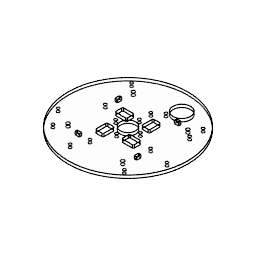
MidPlate_v76 (Autodesk Fusion 360 design; units mm, degrees)
Autodesk Fusion 360 part; units mm, degrees
note: some values were not read from the file. Set by a fixed rule: which face or edge a step refers to.
derive "Sketch1" from "ServoRail v52"
sketch "sketch 220" plane through (0, 0, 0) normal (0, 0, 1) x (1, 0, 0)
  line L0 (-23.75, 13.75) -> (23.75, 13.75) construction
  line L1 (23.75, 13.75) -> (23.75, -13.75) construction
  line L2 (23.75, -13.75) -> (-23.75, -13.75) construction
  line L3 (-23.75, -13.75) -> (-23.75, 13.75) construction
  line L4 (-23.75, 13.75) -> (23.75, -13.75) construction
  line L5 (23.75, 13.75) -> (-23.75, -13.75) construction
  line L6 (-2.75, -24.75) -> (-44.75, -24.75)
  line L7 (-44.75, -24.75) -> (-44.75, -2.75)
  line L8 (-44.75, -2.75) -> (-2.75, -2.75)
  line L9 (-2.75, -2.75) -> (-2.75, -24.75)
  line L10 (-2.75, -24.75) -> (-44.75, -2.75) construction
  line L11 (-44.75, -24.75) -> (-2.75, -2.75) construction
  line L12 (-32.75, -2.75) -> (-32.75, 4.25)
  line L13 (-32.75, 4.25) -> (-29.75, 4.25)
  line L14 (-29.75, 4.25) -> (-29.75, 0.25)
  line L15 (-26.75, 0.25) -> (-26.75, -2.75)
  line L16 (-26.75, 0.25) -> (-29.75, 0.25)
  line L17 (2.75, -44.75) -> (2.75, -2.75)
  line L18 (2.75, -32.75) -> (-4.25, -32.75)
  line L19 (-4.25, -32.75) -> (-4.25, -29.75)
  line L20 (-4.25, -29.75) -> (-0.25, -29.75)
  line L21 (-0.25, -26.75) -> (-0.25, -29.75)
  line L22 (-0.25, -26.75) -> (2.75, -26.75)
  line L23 (24.75, -44.75) -> (2.75, -44.75)
  line L24 (24.75, -2.75) -> (24.75, -44.75)
  line L25 (2.75, -2.75) -> (24.75, -2.75)
  line L26 (44.75, 2.75) -> (2.75, 2.75)
  line L27 (32.75, 2.75) -> (32.75, -4.25)
  line L28 (32.75, -4.25) -> (29.75, -4.25)
  line L29 (29.75, -4.25) -> (29.75, -0.25)
  line L30 (26.75, -0.25) -> (29.75, -0.25)
  line L31 (26.75, -0.25) -> (26.75, 2.75)
  line L32 (44.75, 24.75) -> (44.75, 2.75)
  line L33 (2.75, 24.75) -> (44.75, 24.75)
  line L34 (2.75, 2.75) -> (2.75, 24.75)
  line L35 (-2.75, 44.75) -> (-2.75, 2.75)
  line L36 (-2.75, 32.75) -> (4.25, 32.75)
  line L37 (4.25, 32.75) -> (4.25, 29.75)
  line L38 (4.25, 29.75) -> (0.25, 29.75)
  line L39 (0.25, 26.75) -> (0.25, 29.75)
  line L40 (0.25, 26.75) -> (-2.75, 26.75)
  line L41 (-24.75, 44.75) -> (-2.75, 44.75)
  line L42 (-24.75, 2.75) -> (-24.75, 44.75)
  line L43 (-2.75, 2.75) -> (-24.75, 2.75)
  line L44 (-0.25, -32.75) -> (-0.25, -35.75)
  line L45 (-0.25, -35.75) -> (-7.25, -35.75)
  line L46 (-7.25, -35.75) -> (-7.25, -26.75)
  line L47 (-7.25, -26.75) -> (-0.25, -26.75)
  line L48 (-26.75, -27.75) -> (-29.75, -27.75)
  line L49 (-29.75, -27.75) -> (-29.75, -24.75)
  line L50 (-26.75, -27.75) -> (-26.75, -31.75)
  line L51 (-26.75, -31.75) -> (-23.75, -31.75)
  line L52 (-23.75, -31.75) -> (-23.75, -24.75)
  line L53 (-29.75, -27.75) -> (-29.75, -34.75)
  line L54 (-29.75, -34.75) -> (-20.75, -34.75)
  line L55 (-20.75, -34.75) -> (-20.75, -27.75)
  line L56 (-20.75, -27.75) -> (-23.75, -27.75)
  line L57 (-20.75, -27.75) -> (-7.25, -27.75)
  line L58 (-20.75, -30.75) -> (-7.25, -30.75)
  line L59 (27.75, -29.75) -> (24.75, -29.75)
  line L60 (27.75, -29.75) -> (34.75, -29.75)
  line L61 (27.75, -26.75) -> (27.75, -29.75)
  line L62 (31.75, -23.75) -> (24.75, -23.75)
  line L63 (27.75, -26.75) -> (31.75, -26.75)
  line L64 (31.75, -26.75) -> (31.75, -23.75)
  line L65 (34.75, -29.75) -> (34.75, -20.75)
  line L66 (34.75, -20.75) -> (27.75, -20.75)
  line L67 (27.75, -20.75) -> (27.75, -23.75)
  line L68 (27.75, -20.75) -> (27.75, -7.25)
  line L69 (30.75, -20.75) -> (30.75, -7.25)
  line L70 (26.75, -7.25) -> (26.75, -0.25)
  line L71 (35.75, -7.25) -> (26.75, -7.25)
  line L72 (35.75, -0.25) -> (35.75, -7.25)
  line L73 (32.75, -0.25) -> (35.75, -0.25)
  line L74 (29.75, 27.75) -> (29.75, 24.75)
  line L75 (29.75, 27.75) -> (29.75, 34.75)
  line L76 (26.75, 27.75) -> (29.75, 27.75)
  line L77 (23.75, 31.75) -> (23.75, 24.75)
  line L78 (26.75, 27.75) -> (26.75, 31.75)
  line L79 (26.75, 31.75) -> (23.75, 31.75)
  line L80 (29.75, 34.75) -> (20.75, 34.75)
  line L81 (20.75, 34.75) -> (20.75, 27.75)
  line L82 (20.75, 27.75) -> (23.75, 27.75)
  line L83 (20.75, 27.75) -> (7.25, 27.75)
  line L84 (20.75, 30.75) -> (7.25, 30.75)
  line L85 (7.25, 26.75) -> (0.25, 26.75)
  line L86 (7.25, 35.75) -> (7.25, 26.75)
  line L87 (0.25, 35.75) -> (7.25, 35.75)
  line L88 (0.25, 32.75) -> (0.25, 35.75)
  line L89 (-27.75, 29.75) -> (-24.75, 29.75)
  line L90 (-27.75, 29.75) -> (-34.75, 29.75)
  line L91 (-27.75, 26.75) -> (-27.75, 29.75)
  line L92 (-31.75, 23.75) -> (-24.75, 23.75)
  line L93 (-27.75, 26.75) -> (-31.75, 26.75)
  line L94 (-31.75, 26.75) -> (-31.75, 23.75)
  line L95 (-34.75, 29.75) -> (-34.75, 20.75)
  line L96 (-34.75, 20.75) -> (-27.75, 20.75)
  line L97 (-27.75, 20.75) -> (-27.75, 23.75)
  line L98 (-27.75, 20.75) -> (-27.75, 7.25)
  line L99 (-30.75, 20.75) -> (-30.75, 7.25)
  line L100 (-26.75, 7.25) -> (-26.75, 0.25)
  line L101 (-35.75, 7.25) -> (-26.75, 7.25)
  line L102 (-35.75, 0.25) -> (-35.75, 7.25)
  line L103 (-32.75, 0.25) -> (-35.75, 0.25)
  circle A0 centre (0, 0) radius 56
  circle A1 centre (-41.3532, 14.4521) radius 9.125
  circle A2 centre (-14.4521, -41.3532) radius 9.125
  circle A3 centre (41.3532, -14.4521) radius 9.125
  circle A4 centre (14.4521, 41.3532) radius 9.125
  circle A5 centre (-41.3532, 14.4521) radius 11.125
  circle A6 centre (-14.4521, -41.3532) radius 11.125
  circle A7 centre (41.3532, -14.4521) radius 11.125
  circle A8 centre (14.4521, 41.3532) radius 11.125
  circle A9 centre (0, 0) radius 58
  line L104 (-41.3532, 14.4521) -> (-41.0042, 25.5716)
  line L105 (-41.3532, 14.4521) -> (-41.3532, 3.3271)
  line L106 (0, 0) -> (-41.3532, 14.4521) construction
  line L107 (-14.4521, -41.3532) -> (-25.5716, -41.0042)
  line L108 (-14.4521, -41.3532) -> (-3.3271, -41.3532)
  line L109 (41.3532, -14.4521) -> (41.0042, -25.5716)
  line L110 (41.3532, -14.4521) -> (41.3532, -3.3271)
  line L111 (14.4521, 41.3532) -> (25.5716, 41.0042)
  line L112 (14.4521, 41.3532) -> (3.3271, 41.3532)
  line L113 (2.75, 24.75) -> (-2.75, 24.75)
  line L114 (24.75, -2.75) -> (24.75, 2.75)
  line L115 (-24.75, 2.75) -> (-24.75, -2.75)
  line L116 (-2.75, -24.75) -> (2.75, -24.75)
  circle A10 centre (-7.9571, -31.4571) radius 1.75
  line L117 (-7.25, -30.75) -> (-7.9571, -31.4571)
  line L118 (-18.75, -31.75) -> (-22.75, -31.75)
  line L119 (-22.75, -31.75) -> (-22.75, -29.75)
  line L120 (-22.75, -29.75) -> (-18.75, -29.75)
  line L121 (-18.75, -29.75) -> (-18.75, -31.75)
  line L122 (-18.75, -31.75) -> (-22.75, -29.75) construction
  line L123 (-22.75, -31.75) -> (-18.75, -29.75) construction
  circle A11 centre (31.4571, -7.9571) radius 1.75
  line L124 (31.75, -22.75) -> (29.75, -22.75)
  line L125 (29.75, -22.75) -> (29.75, -18.75)
  line L126 (29.75, -18.75) -> (31.75, -18.75)
  line L127 (31.75, -18.75) -> (31.75, -22.75)
  circle A12 centre (7.9571, 31.4571) radius 1.75
  line L128 (22.75, 31.75) -> (22.75, 29.75)
  line L129 (22.75, 29.75) -> (18.75, 29.75)
  line L130 (18.75, 29.75) -> (18.75, 31.75)
  line L131 (18.75, 31.75) -> (22.75, 31.75)
  circle A13 centre (-31.4571, 7.9571) radius 1.75
  line L132 (-31.75, 22.75) -> (-29.75, 22.75)
  line L133 (-29.75, 22.75) -> (-29.75, 18.75)
  line L134 (-29.75, 18.75) -> (-31.75, 18.75)
  line L135 (-31.75, 18.75) -> (-31.75, 22.75)
  line L136 (29.75, 27.75) -> (33.8506, 28.3482) construction
  circle A14 centre (33.8506, 28.3482) radius 1.75
  circle A15 centre (-28.3482, 33.8506) radius 1.75
  circle A16 centre (-33.8506, -28.3482) radius 1.75
  circle A17 centre (28.3482, -33.8506) radius 1.75
  line L137 (-6.25, -7.75) -> (-14.25, -7.75)
  line L138 (-14.25, -7.75) -> (-14.25, -19.75)
  line L139 (-14.25, -19.75) -> (-6.25, -19.75)
  line L140 (-6.25, -19.75) -> (-6.25, -7.75)
  line L141 (-6.25, -7.75) -> (-14.25, -19.75) construction
  line L142 (-14.25, -7.75) -> (-6.25, -19.75) construction
  line L143 (19.75, -14.25) -> (19.75, -6.25)
  line L144 (7.75, -14.25) -> (19.75, -14.25)
  line L145 (19.75, -6.25) -> (7.75, -6.25)
  line L146 (7.75, -6.25) -> (7.75, -14.25)
  line L147 (14.25, 19.75) -> (6.25, 19.75)
  line L148 (14.25, 7.75) -> (14.25, 19.75)
  line L149 (6.25, 19.75) -> (6.25, 7.75)
  line L150 (6.25, 7.75) -> (14.25, 7.75)
  line L151 (-19.75, 14.25) -> (-19.75, 6.25)
  line L152 (-7.75, 14.25) -> (-19.75, 14.25)
  line L153 (-19.75, 6.25) -> (-7.75, 6.25)
  line L154 (-7.75, 6.25) -> (-7.75, 14.25)
  spline S0 degree 5 poles (-3.3271, -41.3532) (-3.3271, -42.1374) (-3.2169, -43.6541) (-2.7212, -45.7746) (-1.5233, -48.3293) (0.3412, -51.1793) (1.6763, -53.2302) (2.3663, -54.6364) (2.6513, -55.5109) (2.75, -55.9324) knots 0 0 0 0 0 0 0.2 0.4 0.6 0.8 1 1 1 1 1 1
  line L155 (-3.3271, -39.4276) -> (-3.3271, -43.2787)
  line L156 (2.5, -54.8649) -> (3, -57)
  line L157 (2.75, -44.75) -> (2.75, -55.9324) construction
  spline S1 degree 3 poles (-5.3271, -41.3532) (-5.3271, -43.6244) (-4.7917, -45.7291) (-3.9986, -47.5464) (-3.0648, -49.6861) (-1.8311, -51.476) (-0.8806, -52.9928) (-0.0937, -54.2485) (0.4782, -55.3083) (0.7178, -56.0783) (0.7516, -56.1872) (0.7797, -56.2904) (0.8027, -56.3885) knots 0 0 0 0 0.303965 0.303965 0.303965 0.661847 0.661847 0.661847 0.958125 0.958125 0.958125 1 1 1 1
  line L158 (0.6913, -55.9957) -> (2.75, -55.9324)
  spline S2 degree 5 poles (41.3532, -3.3271) (42.1374, -3.3271) (43.6541, -3.2169) (45.7746, -2.7212) (48.3293, -1.5233) (51.1793, 0.3412) (53.2302, 1.6763) (54.6364, 2.3663) (55.5109, 2.6513) (55.9324, 2.75) knots 0 0 0 0 0 0 0.2 0.4 0.6 0.8 1 1 1 1 1 1
  spline S3 degree 3 poles (41.3532, -5.3271) (43.6244, -5.3271) (45.7291, -4.7917) (47.5464, -3.9986) (49.6861, -3.0648) (51.476, -1.8311) (52.9928, -0.8806) (54.2485, -0.0937) (55.3083, 0.4782) (56.0783, 0.7178) (56.1872, 0.7516) (56.2904, 0.7797) (56.3885, 0.8027) knots 0 0 0 0 0.303965 0.303965 0.303965 0.661847 0.661847 0.661847 0.958125 0.958125 0.958125 1 1 1 1
  line L159 (55.9957, 0.6913) -> (55.9324, 2.75)
  spline S4 degree 5 poles (3.3271, 41.3532) (3.3271, 42.1374) (3.2169, 43.6541) (2.7212, 45.7746) (1.5233, 48.3293) (-0.3412, 51.1793) (-1.6763, 53.2302) (-2.3663, 54.6364) (-2.6513, 55.5109) (-2.75, 55.9324) knots 0 0 0 0 0 0 0.2 0.4 0.6 0.8 1 1 1 1 1 1
  spline S5 degree 3 poles (5.3271, 41.3532) (5.3271, 43.6244) (4.7917, 45.7291) (3.9986, 47.5464) (3.0648, 49.6861) (1.8311, 51.476) (0.8806, 52.9928) (0.0937, 54.2485) (-0.4782, 55.3083) (-0.7178, 56.0783) (-0.7516, 56.1872) (-0.7797, 56.2904) (-0.8027, 56.3885) knots 0 0 0 0 0.303965 0.303965 0.303965 0.661847 0.661847 0.661847 0.958125 0.958125 0.958125 1 1 1 1
  line L160 (-0.6913, 55.9957) -> (-2.75, 55.9324)
  spline S6 degree 5 poles (-41.3532, 3.3271) (-42.1374, 3.3271) (-43.6541, 3.2169) (-45.7746, 2.7212) (-48.3293, 1.5233) (-51.1793, -0.3412) (-53.2302, -1.6763) (-54.6364, -2.3663) (-55.5109, -2.6513) (-55.9324, -2.75) knots 0 0 0 0 0 0 0.2 0.4 0.6 0.8 1 1 1 1 1 1
  spline S7 degree 3 poles (-41.3532, 5.3271) (-43.6244, 5.3271) (-45.7291, 4.7917) (-47.5464, 3.9986) (-49.6861, 3.0648) (-51.476, 1.8311) (-52.9928, 0.8806) (-54.2485, 0.0937) (-55.3083, -0.4782) (-56.0783, -0.7178) (-56.1872, -0.7516) (-56.2904, -0.7797) (-56.3885, -0.8027) knots 0 0 0 0 0.303965 0.303965 0.303965 0.661847 0.661847 0.661847 0.958125 0.958125 0.958125 1 1 1 1
  line L161 (-55.9957, -0.6913) -> (-55.9324, -2.75)
  line L162 (-29.75, -34.75) -> (-37.9688, -34.75)
  line L163 (-29.75, -32.75) -> (-38, -32.75)
  spline S8 degree 5 poles (-37.9688, -34.75) (-38.3782, -34.75) (-39.1998, -34.6725) (-40.4402, -34.3239) (-42.1078, -33.4585) (-44.2076, -31.9324) (-45.8949, -30.4934) (-47.1632, -29.3318) (-48.0099, -28.5231) (-48.4336, -28.1103) knots 0 0 0 0 0 0 0.2 0.4 0.6 0.8 1 1 1 1 1 1
  line L164 (-37, -34.75) -> (-38.9375, -34.75)
  spline S9 degree 3 poles (-37.9688, -32.75) (-38.6389, -32.75) (-39.3828, -32.5469) (-40.2776, -32.0885) (-41.7597, -31.3293) (-43.513, -29.9305) (-45.2704, -28.34) (-45.8565, -27.8096) (-46.4464, -27.2542) (-47.0377, -26.678) knots 0 0 0 0 0.31167 0.31167 0.31167 0.827845 0.827845 0.827845 1 1 1 1
  line L165 (-48.4336, -28.1103) -> (-47.0377, -26.678)
  line L166 (34.75, -29.75) -> (34.75, -37.9688)
  line L167 (32.75, -29.75) -> (32.75, -38)
  spline S10 degree 3 poles (32.75, -37.9688) (32.75, -38.6389) (32.5469, -39.3828) (32.0885, -40.2776) (31.3293, -41.7597) (29.9305, -43.513) (28.34, -45.2704) (27.8096, -45.8565) (27.2542, -46.4464) (26.678, -47.0377) knots 0 0 0 0 0.31167 0.31167 0.31167 0.827845 0.827845 0.827845 1 1 1 1
  spline S11 degree 5 poles (34.75, -37.9688) (34.75, -38.3782) (34.6725, -39.1998) (34.3239, -40.4402) (33.4585, -42.1078) (31.9324, -44.2076) (30.4934, -45.8949) (29.3318, -47.1632) (28.5231, -48.0099) (28.1103, -48.4336) knots 0 0 0 0 0 0 0.2 0.4 0.6 0.8 1 1 1 1 1 1
  line L168 (28.1103, -48.4336) -> (26.678, -47.0377)
  line L169 (29.75, 34.75) -> (37.9688, 34.75)
  line L170 (29.75, 32.75) -> (38, 32.75)
  spline S12 degree 3 poles (37.9688, 32.75) (38.6389, 32.75) (39.3828, 32.5469) (40.2776, 32.0885) (41.7597, 31.3293) (43.513, 29.9305) (45.2704, 28.34) (45.8565, 27.8096) (46.4464, 27.2542) (47.0377, 26.678) knots 0 0 0 0 0.31167 0.31167 0.31167 0.827845 0.827845 0.827845 1 1 1 1
  spline S13 degree 5 poles (37.9688, 34.75) (38.3782, 34.75) (39.1998, 34.6725) (40.4402, 34.3239) (42.1078, 33.4585) (44.2076, 31.9324) (45.8949, 30.4934) (47.1632, 29.3318) (48.0099, 28.5231) (48.4336, 28.1103) knots 0 0 0 0 0 0 0.2 0.4 0.6 0.8 1 1 1 1 1 1
  line L171 (48.4336, 28.1103) -> (47.0377, 26.678)
  line L172 (-34.75, 29.75) -> (-34.75, 37.9688)
  line L173 (-32.75, 29.75) -> (-32.75, 38)
  spline S14 degree 3 poles (-32.75, 37.9688) (-32.75, 38.6389) (-32.5469, 39.3828) (-32.0885, 40.2776) (-31.3293, 41.7597) (-29.9305, 43.513) (-28.34, 45.2704) (-27.8096, 45.8565) (-27.2542, 46.4464) (-26.678, 47.0377) knots 0 0 0 0 0.31167 0.31167 0.31167 0.827845 0.827845 0.827845 1 1 1 1
  spline S15 degree 5 poles (-34.75, 37.9688) (-34.75, 38.3782) (-34.6725, 39.1998) (-34.3239, 40.4402) (-33.4585, 42.1078) (-31.9324, 44.2076) (-30.4934, 45.8949) (-29.3318, 47.1632) (-28.5231, 48.0099) (-28.1103, 48.4336) knots 0 0 0 0 0 0 0.2 0.4 0.6 0.8 1 1 1 1 1 1
  line L174 (-28.1103, 48.4336) -> (-26.678, 47.0377)
  point P0 (-23.75, -13.75)
  point P1 (-20.75, -30.75)
  point P2 (-10.25, -13.75)
extrude "Extrude1" add sketch "sketch 220" along normal blind 3 contours L6 L17 L22 L46 L47 L52 L56 L57 L116 | L6 L7 L8 L9 | L8 L9 L17 L25 L26 L34 L35 L43 L113 L114 L115 L116 | L6 L48 L49 L50 L51 L52 | L17 L23 L24 L25 | L6 L7 L8 L12 L49 L53 L102 L103 A0 A5 S6 L163 S9 L165 | L48 L50 L51 L52 L53 L54 L55 L56 A6 L118 L119 L120 | L8 L15 L42 L92 L97 L98 L100 L101 L115 | L17 L18 L19 L20 L21 L22 | L46 L55 L57 L58 A6 A10 L120 L121 | L8 L12 L13 L14 L15 L16 | L35 L41 L42 L43 | L17 L18 L23 L24 L44 L45 L59 L60 A0 A6 S0 L167 S10 L168 | L18 L19 L20 L21 L44 L45 L46 L47 A6 A10 | L24 L26 L31 L62 L67 L68 L70 L71 L114 | L53 L162 L163 S8 L164 S9 L165 | L12 L13 L14 L16 L100 L101 L102 L103 A5 A13 | L42 L89 L91 L92 L93 L94 | L24 L59 L61 L62 L63 L64 | L26 L32 L33 L34 | L54 A0 A6 S1 L162 S8 L164 | L35 L36 L41 L42 L87 L88 L89 L90 A0 A8 S4 L173 S14 L174 | L90 L91 L92 L93 L94 L95 L96 L97 A5 L132 L133 L135 | L33 L35 L40 L77 L82 L83 L85 L86 L113 | L60 L61 L62 L63 L64 L65 L66 L67 A7 L124 L125 L127 | L26 L27 L28 L29 L30 L31 | L54 L55 A6 | L54 A2 A6 L107 | L55 A6 L118 | L58 A6 L121 | L58 A6 A10 | L96 L98 L99 L101 A5 A13 L133 L134 | L35 L36 L37 L38 L39 L40 | L45 A2 A6 L108 | L45 L46 A6 A10 | L66 L68 L69 L71 A7 A11 L125 L126 | L26 L27 L32 L33 L72 L73 L74 L75 A0 A7 S2 L170 S12 L171 | L27 L28 L29 L30 L70 L71 L72 L73 A7 A11 | L46 L55 L58 A2 A6 A10 L118 L121 | A2 L107 L108 | A2 A6 L107 S1 | L58 A6 | L102 A1 A5 L105 | L101 L102 A5 A13 | L90 L172 L173 S14 S15 L174 | L36 L37 L38 L39 L85 L86 L87 L88 A8 A12 | L33 L74 L76 L77 L78 L79 | A6 S0 S1 L158 | A6 L108 S1 | L60 L166 L167 S10 S11 L168 | A2 L107 L108 | L96 L99 L101 A1 A5 A13 L134 L135 | A1 L104 L105 | A5 S6 S7 L161 | A5 L105 S7 | L95 A0 A5 S7 L172 S15 | L75 L76 L77 L78 L79 L80 L81 L82 A8 L128 L129 L131 | A0 L158 | L65 A0 A7 S3 L166 S11 | A0 L161 | A1 A5 L104 S7 | A1 L104 L105 | L99 A5 A13 | L95 L96 A5 | L95 A1 A5 L104 | L96 A5 L135 | L99 A5 L134 | L81 L83 L84 L86 A8 A12 L129 L130 | L65 L66 A7 | L65 A3 A7 L109 | L66 A7 L127 | L69 A7 L126 | L71 L72 A7 A11 | L69 A7 A11 | L72 A3 A7 L110 | L99 A5 | L87 A4 A8 L112 | L86 L87 A8 A12 | L75 L169 L170 S12 S13 L171 | L66 L69 L71 A3 A7 A11 L126 L127 | A3 L109 L110 | A3 A7 L109 S3 | L69 A7 | A7 S2 S3 L159 | A7 L110 S3 | A8 S4 S5 L160 | A0 L160 | L81 L84 L86 A4 A8 A12 L130 L131 | A8 L112 S5 | L84 A8 A12 | L80 A0 A8 S5 L169 S13 | A0 L159 | A3 L109 L110 | A4 A8 L111 S5 | L80 A4 A8 L111 | L80 L81 A8 | L84 A8 | L81 A8 L131 | L84 A8 L130
move_face "OffsetFaces1" offset 0.25 24 faces at (-6.3777, -32.2107, 2) (-7.1741, -33.0221, 2) (-9.5317, -32.2208, 2) (-9.6584, -31.0469, 2) (-9.1804, -30.2057, 2) (-6.3352, -30.8, 2) (-31.8536, 6.2526, 2) (-32.999, 7.1293, 2) (-31.9794, 9.6274, 2) (-31.0469, 9.6584, 2) (-29.9466, 8.8407, 2) (-29.7146, 7.7956, 2) (6.5889, 32.5483, 2) (7.1293, 32.999, 2) (9.3372, 32.5332, 2) (9.707, 31.439, 2) (9.6926, 31.232, 2) (8.6277, 29.8407, 2) (32.101, -6.3299, 2) (33.051, -7.2347, 1) (33.1606, -7.5563, 2) (32.3777, -9.4454, 2) (31.232, -9.6926, 2) (30.6746, -9.5224, 2)
move_face "OffsetFaces2" offset -0.2 36 faces at (-19.1895, -31.75, 1) (-20.2957, -31.75, 1) (-21.4167, -31.75, 1) (-18.75, -30.0833, 1) (-18.75, -30.864, 1) (-18.75, -31.3113, 1) (31.0833, -22.75, 1) (31.75, -19.1895, 1) (31.75, -20.2957, 1) (31.75, -21.4167, 1) (22.0833, 29.75, 1) (20.0833, 29.75, 1) (22.75, 31.0833, 2) (19.1895, 31.75, 1) (20.2957, 31.75, 1) (21.4167, 31.75, 1) (18.75, 30.0833, 1) (18.75, 30.864, 1) (18.75, 31.3113, 1) (30.0833, -18.75, 1) (30.864, -18.75, 1) (31.3113, -18.75, 1) (29.75, -22.0833, 1) (29.75, -20.0833, 1) (-20.0833, -29.75, 1) (-22.0833, -29.75, 1) (-22.75, -31.0833, 1) (-31.0833, 22.75, 2) (-31.75, 19.1895, 1) (-31.75, 20.2957, 1) (-31.75, 21.4167, 1) (-29.75, 22.0833, 1) (-29.75, 20.0833, 1) (-30.0833, 18.75, 1) (-30.864, 18.75, 1) (-31.3113, 18.75, 1)
derive "Sketch3" from "MiddleSupport v33"
sketch "sketch 1885" plane through (0, 0, 0) normal (0, 0, 1) x (1, 0, 0)
  circle A0 centre (0, 0) radius 4
  circle A1 centre (0, 0) radius 1
  line L0 (15, 0) -> (0, 0)
  line L1 (0, 0) -> (0, 2)
  line L2 (0, 2) -> (15, 2)
  line L3 (15, 2) -> (15, 0)
  line L4 (0, 15) -> (0, 0)
  line L5 (-2, 15) -> (0, 15)
  line L6 (-2, 0) -> (-2, 15)
  line L7 (0, 0) -> (-2, 0)
  line L8 (-15, 0) -> (0, 0)
  line L9 (-15, -2) -> (-15, 0)
  line L10 (0, -2) -> (-15, -2)
  line L11 (0, 0) -> (0, -2)
  line L12 (0, -15) -> (0, 0)
  line L13 (2, -15) -> (0, -15)
  line L14 (2, 0) -> (2, -15)
  line L15 (0, 0) -> (2, 0)
  circle A2 centre (0, 0) radius 10
  circle A3 centre (12.2939, 0.4894) radius 1.75
  circle A4 centre (12.2939, 0.4894) radius 2.75
  circle A5 centre (-0.4894, 12.2939) radius 2.75
  circle A6 centre (-0.4894, 12.2939) radius 1.75
  circle A7 centre (-12.2939, -0.4894) radius 2.75
  circle A8 centre (-12.2939, -0.4894) radius 1.75
  circle A9 centre (0.4894, -12.2939) radius 2.75
  circle A10 centre (0.4894, -12.2939) radius 1.75
  circle A11 centre (0, 0) radius 8
extrude "Extrude3" cut sketch "sketch 1885" along normal blind 2 contours A0 A1 L0 L1 L2 L4 L15 | A0 L0 L14 A11 | A0 L0 L2 A11 | A0 L0 L14 | A0 L2 L4 | A0 L2 L4 A11 | A0 L12 L14 A11 | A0 A1 L0 L11 L12 L14 L15 | A0 A1 L1 L4 L6 L7 L8 | A0 L4 L6 A11 | A0 L10 L12 A11 | A0 L10 L12 | A1 L0 L1 L4 L15 | A1 L0 L11 L12 L15 | A0 L6 L8 | A0 L6 L8 A11 | A1 L1 L4 L7 L8 | A0 L8 L10 A11 | A0 A1 L7 L8 L10 L11 L12 | A1 L7 L8 L11 L12 | L0 L2 A3 | L0 A3 | L2 A3 | L14 A10 | L12 L14 A10 | L4 L6 A6 | L4 A6 | L12 A10 | L6 A6 | L10 A8 | L8 L10 A8 | L8 A8
move_face "OffsetFaces3" offset 0.25 4 faces at (-10.5526, -0.3152, 1.3333) (1.2519, 12.4681, 1.3333) (14.0417, 0.4022, 0.6667) (2.2372, -12.3811, 0.6667)
move_face "OffsetFaces5" offset 6 1 faces at (-55.9304, 2.7914, 1)
derive "Sketch2" from "OuterShellUpper v68"
fillet "Fillet1" radius 1 16 edges at (-14.25, -19.75, 1.5) (-6.25, -19.75, 1.5) (-14.25, -7.75, 1.5) (-6.25, -7.75, 1.5) (7.75, -14.25, 1.5) (19.75, -14.25, 1.5) (7.75, -6.25, 1.5) (19.75, -6.25, 1.5) (6.25, 19.75, 1.5) (6.25, 7.75, 1.5) (14.25, 7.75, 1.5) (14.25, 19.75, 1.5) (-19.75, 6.25, 1.5) (-7.75, 6.25, 1.5) (-7.75, 14.25, 1.5) (-19.75, 14.25, 1.5)
sketch "Sketch4" plane through (0, 0, 0) normal (0, 0, -1) x (1, 0, 0)
  circle A0 centre (-0.4894, -12.2939) radius 1.5
  circle A1 centre (12.2939, -0.4894) radius 1.5
  circle A2 centre (-12.2939, 0.4894) radius 1.5
  circle A3 centre (0.4894, 12.2939) radius 1.5
  circle A4 centre (0, 0) radius 8
  arc A5 (-7.25, 7.75) -> (-6.25, 8.75) centre (-7.25, 8.75) ccw
  line L0 (-7.25, 7.75) -> (-13.25, 7.75)
  arc A6 (-14.25, 8.75) -> (-13.25, 7.75) centre (-13.25, 8.75) ccw
  line L1 (-14.25, 8.75) -> (-14.25, 18.75)
  arc A7 (-13.25, 19.75) -> (-14.25, 18.75) centre (-13.25, 18.75) ccw
  line L2 (-13.25, 19.75) -> (-7.25, 19.75)
  arc A8 (-6.25, 18.75) -> (-7.25, 19.75) centre (-7.25, 18.75) ccw
  line L3 (-6.25, 18.75) -> (-6.25, 8.75)
  line L4 (31.95, 18.55) -> (29.55, 18.55)
  line L5 (29.55, 18.55) -> (29.55, 22.95)
  line L6 (29.55, 22.95) -> (31.95, 22.95)
  line L7 (31.95, 22.95) -> (31.95, 18.55)
  circle A9 centre (-33.8506, 28.3482) radius 1.75
  circle A10 centre (-31.4571, -7.9571) radius 1.5
  circle A11 centre (28.3482, 33.8506) radius 1.75
  arc A12 (-8.75, -14.25) -> (-7.75, -13.25) centre (-8.75, -13.25) ccw
  line L8 (-8.75, -14.25) -> (-18.75, -14.25)
  arc A13 (-19.75, -13.25) -> (-18.75, -14.25) centre (-18.75, -13.25) ccw
  line L9 (-19.75, -13.25) -> (-19.75, -7.25)
  arc A14 (-18.75, -6.25) -> (-19.75, -7.25) centre (-18.75, -7.25) ccw
  line L10 (-18.75, -6.25) -> (-8.75, -6.25)
  arc A15 (-7.75, -7.25) -> (-8.75, -6.25) centre (-8.75, -7.25) ccw
  line L11 (-7.75, -7.25) -> (-7.75, -13.25)
  circle A16 centre (-7.9571, 31.4571) radius 1.5
  line L12 (-31.95, -18.55) -> (-29.55, -18.55)
  line L13 (-29.55, -18.55) -> (-29.55, -22.95)
  line L14 (-29.55, -22.95) -> (-31.95, -22.95)
  line L15 (-31.95, -22.95) -> (-31.95, -18.55)
  circle A17 centre (7.9571, -31.4571) radius 1.5
  circle A18 centre (31.4571, 7.9571) radius 1.5
  circle A19 centre (14.4521, -41.3532) radius 9.125
  line L16 (18.55, -31.95) -> (18.55, -29.55)
  line L17 (18.55, -29.55) -> (22.95, -29.55)
  line L18 (22.95, -29.55) -> (22.95, -31.95)
  line L19 (22.95, -31.95) -> (18.55, -31.95)
  circle A20 centre (0, 0) radius 62
  line L20 (-18.55, 29.55) -> (-22.95, 29.55)
  line L21 (-22.95, 29.55) -> (-22.95, 31.95)
  line L22 (-22.95, 31.95) -> (-18.55, 31.95)
  line L23 (-18.55, 31.95) -> (-18.55, 29.55)
  circle A21 centre (-28.3482, -33.8506) radius 1.75
  arc A22 (14.25, -8.75) -> (13.25, -7.75) centre (13.25, -8.75) ccw
  line L24 (14.25, -8.75) -> (14.25, -18.75)
  arc A23 (13.25, -19.75) -> (14.25, -18.75) centre (13.25, -18.75) ccw
  line L25 (13.25, -19.75) -> (7.25, -19.75)
  arc A24 (6.25, -18.75) -> (7.25, -19.75) centre (7.25, -18.75) ccw
  line L26 (6.25, -18.75) -> (6.25, -8.75)
  arc A25 (7.25, -7.75) -> (6.25, -8.75) centre (7.25, -8.75) ccw
  line L27 (7.25, -7.75) -> (13.25, -7.75)
  circle A26 centre (33.8506, -28.3482) radius 1.75
  arc A27 (8.75, 14.25) -> (7.75, 13.25) centre (8.75, 13.25) ccw
  line L28 (8.75, 14.25) -> (18.75, 14.25)
  arc A28 (19.75, 13.25) -> (18.75, 14.25) centre (18.75, 13.25) ccw
  line L29 (19.75, 13.25) -> (19.75, 7.25)
  arc A29 (18.75, 6.25) -> (19.75, 7.25) centre (18.75, 7.25) ccw
  line L30 (18.75, 6.25) -> (8.75, 6.25)
  arc A30 (7.75, 7.25) -> (8.75, 6.25) centre (8.75, 7.25) ccw
  line L31 (7.75, 7.25) -> (7.75, 13.25)
  circle A31 centre (-18.283, 13.9511) radius 3
  circle A32 centre (-18.283, 13.9511) radius 1.5
  line L32 (-18.283, 13.9511) -> (-16.0069, 35.2598) construction
  line L33 (-43.7745, 4.226) -> (-18.283, 13.9511) construction
  circle A33 centre (-43.7745, 4.226) radius 3
  circle A34 centre (-43.7745, 4.226) radius 1.5
  line L34 (-16.0069, 35.2598) -> (-43.7745, 4.226) construction
  circle A35 centre (-16.0069, 35.2598) radius 3
  circle A36 centre (-16.0069, 35.2598) radius 1.5
  circle A37 centre (36.1331, 14.7602) radius 1.5
  circle A38 centre (22.7515, 18.8754) radius 1.5
  circle A39 centre (17.5503, -13.7122) radius 1.5
  line L35 (36.1331, 14.7602) -> (22.7515, 18.8754) construction
  line L36 (22.7515, 18.8754) -> (17.5503, -13.7122) construction
  line L37 (17.5503, -13.7122) -> (36.1331, 14.7602) construction
  circle A40 centre (4.5537, -49.7247) radius 1.5
  line L38 (-4.2969, -53.5838) -> (-2.7827, -51.7218)
  line L39 (-2.7827, -51.7218) -> (-7.7482, -47.684)
  line L40 (-7.7482, -47.684) -> (-9.2624, -49.546)
  line L41 (-9.2624, -49.546) -> (-4.2969, -53.5838)
  dimension "d37" = 3
  dimension "d38" = 6
  dimension "d39" = 3
  dimension "d40" = 6
  dimension "d41" = 3
  dimension "d42" = 6
  dimension "d45" = 21.4299
  dimension "d49" = 3
  dimension "d50" = 3
  dimension "d51" = 3
  dimension "d52" = 14
  dimension "d53" = 33
  dimension "d54" = 34
  dimension "d57" = 3
  dimension "d58" = 2.4
  dimension "d59" = 6.4
  constraint concentric A35 A36
  constraint concentric A33 A34
  constraint concentric A31 A32
  constraint coincident L32.end L34.start
  constraint coincident L33.start A33.centre
  constraint coincident A31.centre A32.centre
  constraint coincident A37.centre L35.start
  constraint coincident A38.centre L35.end
  constraint coincident A39.centre L36.end
  constraint perpendicular L38 L39
  constraint parallel L38 L40
  constraint parallel L39 L41
  measures "d37" diameter of A36
  measures "d38" diameter of A35
  measures "d39" diameter of A34
  measures "d40" diameter of A33
  measures "d41" diameter of A32
  measures "d42" diameter of A31
  measures "d45" distance of A31.centre L32.end
  measures "d49" diameter of A37
  measures "d50" diameter of A38
  measures "d51" diameter of A39
  measures "d52" distance of A37.centre A38.centre
  measures "d53" distance of A38.centre A39.centre
  measures "d54" distance of A37.centre A39.centre
  measures "d57" diameter of A40
  measures "d58" distance of L38.start L38.end
  measures "d59" distance of L38.start L40.end
sketch "Sketch6" plane through (0, 0, 3) normal (0, 0, 1) x (-1, 0, 0)
  line L0 (6.25, 8.75) -> (6.25, 18.75)
  arc A0 (7.25, 19.75) -> (6.25, 18.75) centre (7.25, 18.75) ccw
  line L1 (7.25, 19.75) -> (13.25, 19.75)
  arc A1 (14.25, 18.75) -> (13.25, 19.75) centre (13.25, 18.75) ccw
  line L2 (14.25, 18.75) -> (14.25, 8.75)
  arc A2 (13.25, 7.75) -> (14.25, 8.75) centre (13.25, 8.75) ccw
  line L3 (13.25, 7.75) -> (7.25, 7.75)
  arc A3 (6.25, 8.75) -> (7.25, 7.75) centre (7.25, 8.75) ccw
  line L4 (-29.55, 18.55) -> (-31.95, 18.55)
  line L5 (-31.95, 18.55) -> (-31.95, 22.95)
  line L6 (-31.95, 22.95) -> (-29.55, 22.95)
  line L7 (-29.55, 22.95) -> (-29.55, 18.55)
  circle A4 centre (33.8506, 28.3482) radius 1.75
  circle A5 centre (31.4571, -7.9571) radius 1.5
  circle A6 centre (-28.3482, 33.8506) radius 1.75
  line L8 (7.75, -13.25) -> (7.75, -7.25)
  arc A7 (8.75, -6.25) -> (7.75, -7.25) centre (8.75, -7.25) ccw
  line L9 (8.75, -6.25) -> (18.75, -6.25)
  arc A8 (19.75, -7.25) -> (18.75, -6.25) centre (18.75, -7.25) ccw
  line L10 (19.75, -7.25) -> (19.75, -13.25)
  arc A9 (18.75, -14.25) -> (19.75, -13.25) centre (18.75, -13.25) ccw
  line L11 (18.75, -14.25) -> (8.75, -14.25)
  arc A10 (7.75, -13.25) -> (8.75, -14.25) centre (8.75, -13.25) ccw
  circle A11 centre (7.9571, 31.4571) radius 1.5
  line L12 (29.55, -18.55) -> (31.95, -18.55)
  line L13 (31.95, -18.55) -> (31.95, -22.95)
  line L14 (31.95, -22.95) -> (29.55, -22.95)
  line L15 (29.55, -22.95) -> (29.55, -18.55)
  circle A12 centre (-7.9571, -31.4571) radius 1.5
  circle A13 centre (-31.4571, 7.9571) radius 1.5
  circle A14 centre (-14.4521, -41.3532) radius 9.125
  line L16 (-18.55, -29.55) -> (-18.55, -31.95)
  line L17 (-18.55, -31.95) -> (-22.95, -31.95)
  line L18 (-22.95, -31.95) -> (-22.95, -29.55)
  line L19 (-22.95, -29.55) -> (-18.55, -29.55)
  circle A15 centre (0, 0) radius 62
  line L20 (22.95, 29.55) -> (18.55, 29.55)
  line L21 (18.55, 29.55) -> (18.55, 31.95)
  line L22 (18.55, 31.95) -> (22.95, 31.95)
  line L23 (22.95, 31.95) -> (22.95, 29.55)
  circle A16 centre (28.3482, -33.8506) radius 1.75
  line L24 (-13.25, -7.75) -> (-7.25, -7.75)
  arc A17 (-6.25, -8.75) -> (-7.25, -7.75) centre (-7.25, -8.75) ccw
  line L25 (-6.25, -8.75) -> (-6.25, -18.75)
  arc A18 (-7.25, -19.75) -> (-6.25, -18.75) centre (-7.25, -18.75) ccw
  line L26 (-7.25, -19.75) -> (-13.25, -19.75)
  arc A19 (-14.25, -18.75) -> (-13.25, -19.75) centre (-13.25, -18.75) ccw
  line L27 (-14.25, -18.75) -> (-14.25, -8.75)
  arc A20 (-13.25, -7.75) -> (-14.25, -8.75) centre (-13.25, -8.75) ccw
  circle A21 centre (-33.8506, -28.3482) radius 1.75
  line L28 (-7.75, 13.25) -> (-7.75, 7.25)
  arc A22 (-8.75, 6.25) -> (-7.75, 7.25) centre (-8.75, 7.25) ccw
  line L29 (-8.75, 6.25) -> (-18.75, 6.25)
  arc A23 (-19.75, 7.25) -> (-18.75, 6.25) centre (-18.75, 7.25) ccw
  line L30 (-19.75, 7.25) -> (-19.75, 13.25)
  arc A24 (-18.75, 14.25) -> (-19.75, 13.25) centre (-18.75, 13.25) ccw
  line L31 (-18.75, 14.25) -> (-8.75, 14.25)
  arc A25 (-7.75, 13.25) -> (-8.75, 14.25) centre (-8.75, 13.25) ccw
sketch "Sketch7" plane through (0, 0, 0) normal (0, 0, -1) x (1, 0, 0)
  circle A0 centre (-0.4894, -12.2939) radius 1.5
  circle A1 centre (12.2939, -0.4894) radius 1.5
  circle A2 centre (-12.2939, 0.4894) radius 1.5
  circle A3 centre (0.4894, 12.2939) radius 1.5
  circle A4 centre (0, 0) radius 8
  circle A5 centre (-33.8506, 28.3482) radius 1.75
  circle A6 centre (-7.9571, 31.4571) radius 1.5
  circle A7 centre (7.9571, -31.4571) radius 1.5
  line L0 (18.55, -31.95) -> (18.55, -29.55)
  line L1 (18.55, -29.55) -> (22.95, -29.55)
  line L2 (22.95, -29.55) -> (22.95, -31.95)
  line L3 (22.95, -31.95) -> (18.55, -31.95)
  line L4 (-18.55, 29.55) -> (-22.95, 29.55)
  line L5 (-22.95, 29.55) -> (-22.95, 31.95)
  line L6 (-22.95, 31.95) -> (-18.55, 31.95)
  line L7 (-18.55, 31.95) -> (-18.55, 29.55)
  circle A8 centre (31.4571, 7.9571) radius 1.5
  arc A9 (14.25, -8.75) -> (13.25, -7.75) centre (13.25, -8.75) ccw
  line L8 (14.25, -8.75) -> (14.25, -18.75)
  arc A10 (13.25, -19.75) -> (14.25, -18.75) centre (13.25, -18.75) ccw
  line L9 (13.25, -19.75) -> (7.25, -19.75)
  arc A11 (6.25, -18.75) -> (7.25, -19.75) centre (7.25, -18.75) ccw
  line L10 (6.25, -18.75) -> (6.25, -8.75)
  arc A12 (7.25, -7.75) -> (6.25, -8.75) centre (7.25, -8.75) ccw
  line L11 (7.25, -7.75) -> (13.25, -7.75)
  circle A13 centre (28.3482, 33.8506) radius 1.75
  arc A14 (-7.25, 7.75) -> (-6.25, 8.75) centre (-7.25, 8.75) ccw
  line L12 (-7.25, 7.75) -> (-13.25, 7.75)
  arc A15 (-14.25, 8.75) -> (-13.25, 7.75) centre (-13.25, 8.75) ccw
  line L13 (-14.25, 8.75) -> (-14.25, 18.75)
  arc A16 (-13.25, 19.75) -> (-14.25, 18.75) centre (-13.25, 18.75) ccw
  line L14 (-13.25, 19.75) -> (-7.25, 19.75)
  arc A17 (-6.25, 18.75) -> (-7.25, 19.75) centre (-7.25, 18.75) ccw
  line L15 (-6.25, 18.75) -> (-6.25, 8.75)
  line L16 (31.95, 18.55) -> (29.55, 18.55)
  line L17 (29.55, 18.55) -> (29.55, 22.95)
  line L18 (29.55, 22.95) -> (31.95, 22.95)
  line L19 (31.95, 22.95) -> (31.95, 18.55)
  circle A18 centre (-31.4571, -7.9571) radius 1.5
  line L20 (-31.95, -18.55) -> (-29.55, -18.55)
  line L21 (-29.55, -18.55) -> (-29.55, -22.95)
  line L22 (-29.55, -22.95) -> (-31.95, -22.95)
  line L23 (-31.95, -22.95) -> (-31.95, -18.55)
  circle A19 centre (0, 0) radius 62
  circle A20 centre (33.8506, -28.3482) radius 1.75
  arc A21 (-8.75, -14.25) -> (-7.75, -13.25) centre (-8.75, -13.25) ccw
  line L24 (-8.75, -14.25) -> (-18.75, -14.25)
  arc A22 (-19.75, -13.25) -> (-18.75, -14.25) centre (-18.75, -13.25) ccw
  line L25 (-19.75, -13.25) -> (-19.75, -7.25)
  arc A23 (-18.75, -6.25) -> (-19.75, -7.25) centre (-18.75, -7.25) ccw
  line L26 (-18.75, -6.25) -> (-8.75, -6.25)
  arc A24 (-7.75, -7.25) -> (-8.75, -6.25) centre (-8.75, -7.25) ccw
  line L27 (-7.75, -7.25) -> (-7.75, -13.25)
  arc A25 (8.75, 14.25) -> (7.75, 13.25) centre (8.75, 13.25) ccw
  line L28 (8.75, 14.25) -> (18.75, 14.25)
  arc A26 (19.75, 13.25) -> (18.75, 14.25) centre (18.75, 13.25) ccw
  line L29 (19.75, 13.25) -> (19.75, 7.25)
  arc A27 (18.75, 6.25) -> (19.75, 7.25) centre (18.75, 7.25) ccw
  line L30 (18.75, 6.25) -> (8.75, 6.25)
  arc A28 (7.75, 7.25) -> (8.75, 6.25) centre (8.75, 7.25) ccw
  line L31 (7.75, 7.25) -> (7.75, 13.25)
  circle A29 centre (-28.3482, -33.8506) radius 1.75
  circle A30 centre (14.4521, -41.3532) radius 9.125
  circle A31 centre (-52.5447, 19.941) radius 1.5
  circle A32 centre (-14, 46) radius 1.5
  circle A33 centre (52.6829, 12.2455) radius 1.5
  circle A34 centre (41, -23) radius 1.5
  circle A35 centre (-0.3626, -24.0582) radius 1.5
  dimension "d60" = 3
  dimension "d61" = 3
  dimension "d63" = 3
  dimension "d64" = 3
  dimension "d65" = 3
  measures "d60" diameter of A31
  measures "d61" diameter of A32
  measures "d63" diameter of A33
  measures "d64" diameter of A34
  measures "d65" diameter of A35
extrude "Extrude8" cut sketch "Sketch7" against normal blind 10 contours A31 | A32 | A33 | A34 | A35
sketch "Sketch9" plane through (0, 0, 0) normal (0, 0, -1) x (1, 0, 0)
  circle A0 centre (-0.4894, -12.2939) radius 1.5
  circle A1 centre (12.2939, -0.4894) radius 1.5
  circle A2 centre (-12.2939, 0.4894) radius 1.5
  circle A3 centre (0.4894, 12.2939) radius 1.5
  circle A4 centre (0, 0) radius 8
  circle A5 centre (-33.8506, 28.3482) radius 1.75
  circle A6 centre (-7.9571, 31.4571) radius 1.5
  circle A7 centre (7.9571, -31.4571) radius 1.5
  line L0 (18.55, -31.95) -> (18.55, -29.55)
  line L1 (18.55, -29.55) -> (22.95, -29.55)
  line L2 (22.95, -29.55) -> (22.95, -31.95)
  line L3 (22.95, -31.95) -> (18.55, -31.95)
  line L4 (-18.55, 29.55) -> (-22.95, 29.55)
  line L5 (-22.95, 29.55) -> (-22.95, 31.95)
  line L6 (-22.95, 31.95) -> (-18.55, 31.95)
  line L7 (-18.55, 31.95) -> (-18.55, 29.55)
  circle A8 centre (31.4571, 7.9571) radius 1.5
  arc A9 (14.25, -8.75) -> (13.25, -7.75) centre (13.25, -8.75) ccw
  line L8 (14.25, -8.75) -> (14.25, -18.75)
  arc A10 (13.25, -19.75) -> (14.25, -18.75) centre (13.25, -18.75) ccw
  line L9 (13.25, -19.75) -> (7.25, -19.75)
  arc A11 (6.25, -18.75) -> (7.25, -19.75) centre (7.25, -18.75) ccw
  line L10 (6.25, -18.75) -> (6.25, -8.75)
  arc A12 (7.25, -7.75) -> (6.25, -8.75) centre (7.25, -8.75) ccw
  line L11 (7.25, -7.75) -> (13.25, -7.75)
  circle A13 centre (28.3482, 33.8506) radius 1.75
  arc A14 (-7.25, 7.75) -> (-6.25, 8.75) centre (-7.25, 8.75) ccw
  line L12 (-7.25, 7.75) -> (-13.25, 7.75)
  arc A15 (-14.25, 8.75) -> (-13.25, 7.75) centre (-13.25, 8.75) ccw
  line L13 (-14.25, 8.75) -> (-14.25, 18.75)
  arc A16 (-13.25, 19.75) -> (-14.25, 18.75) centre (-13.25, 18.75) ccw
  line L14 (-13.25, 19.75) -> (-7.25, 19.75)
  arc A17 (-6.25, 18.75) -> (-7.25, 19.75) centre (-7.25, 18.75) ccw
  line L15 (-6.25, 18.75) -> (-6.25, 8.75)
  line L16 (31.95, 18.55) -> (29.55, 18.55)
  line L17 (29.55, 18.55) -> (29.55, 22.95)
  line L18 (29.55, 22.95) -> (31.95, 22.95)
  line L19 (31.95, 22.95) -> (31.95, 18.55)
  circle A18 centre (-31.4571, -7.9571) radius 1.5
  line L20 (-31.95, -18.55) -> (-29.55, -18.55)
  line L21 (-29.55, -18.55) -> (-29.55, -22.95)
  line L22 (-29.55, -22.95) -> (-31.95, -22.95)
  line L23 (-31.95, -22.95) -> (-31.95, -18.55)
  circle A19 centre (0, 0) radius 62
  circle A20 centre (33.8506, -28.3482) radius 1.75
  arc A21 (-8.75, -14.25) -> (-7.75, -13.25) centre (-8.75, -13.25) ccw
  line L24 (-8.75, -14.25) -> (-18.75, -14.25)
  arc A22 (-19.75, -13.25) -> (-18.75, -14.25) centre (-18.75, -13.25) ccw
  line L25 (-19.75, -13.25) -> (-19.75, -7.25)
  arc A23 (-18.75, -6.25) -> (-19.75, -7.25) centre (-18.75, -7.25) ccw
  line L26 (-18.75, -6.25) -> (-8.75, -6.25)
  arc A24 (-7.75, -7.25) -> (-8.75, -6.25) centre (-8.75, -7.25) ccw
  line L27 (-7.75, -7.25) -> (-7.75, -13.25)
  arc A25 (8.75, 14.25) -> (7.75, 13.25) centre (8.75, 13.25) ccw
  line L28 (8.75, 14.25) -> (18.75, 14.25)
  arc A26 (19.75, 13.25) -> (18.75, 14.25) centre (18.75, 13.25) ccw
  line L29 (19.75, 13.25) -> (19.75, 7.25)
  arc A27 (18.75, 6.25) -> (19.75, 7.25) centre (18.75, 7.25) ccw
  line L30 (18.75, 6.25) -> (8.75, 6.25)
  arc A28 (7.75, 7.25) -> (8.75, 6.25) centre (8.75, 7.25) ccw
  line L31 (7.75, 7.25) -> (7.75, 13.25)
  circle A29 centre (-28.3482, -33.8506) radius 1.75
  circle A30 centre (14.4521, -41.3532) radius 9.125
  circle A31 centre (-0.3626, -24.0582) radius 1.5
  circle A32 centre (-14, 46) radius 1.5
  circle A33 centre (41, -23) radius 1.5
  circle A34 centre (-52.5447, 19.941) radius 1.5
  circle A35 centre (52.6829, 12.2455) radius 1.5
  circle A36 centre (-40.8377, 37.077) radius 1.5
  circle A37 centre (-37.077, -40.8377) radius 1.5
  circle A38 centre (40.8377, -37.077) radius 1.5
  circle A39 centre (37.077, 40.8377) radius 1.5
  dimension "d68" = 3
  dimension "d70" = 360
  measures "d68" diameter of A36
extrude "Extrude9" cut sketch "Sketch9" against normal blind 11 contours A36 | A37 | A38 | A39
sketch "Sketch10" plane through (0, 0, 3) normal (0, 0, 1) x (-1, 0, 0)
  circle A0 centre (-52.6829, 12.2455) radius 1.5
  circle A1 centre (14, 46) radius 1.5
  circle A2 centre (-41, -23) radius 1.5
  circle A3 centre (52.5447, 19.941) radius 1.5
  circle A4 centre (0.3626, -24.0582) radius 1.5
  circle A5 centre (-14.4521, -41.3532) radius 9.125
  circle A6 centre (28.3482, -33.8506) radius 1.75
  line L0 (-7.75, 13.25) -> (-7.75, 7.25)
  arc A7 (-8.75, 6.25) -> (-7.75, 7.25) centre (-8.75, 7.25) ccw
  line L1 (-8.75, 6.25) -> (-18.75, 6.25)
  arc A8 (-19.75, 7.25) -> (-18.75, 6.25) centre (-18.75, 7.25) ccw
  line L2 (-19.75, 7.25) -> (-19.75, 13.25)
  arc A9 (-18.75, 14.25) -> (-19.75, 13.25) centre (-18.75, 13.25) ccw
  line L3 (-18.75, 14.25) -> (-8.75, 14.25)
  arc A10 (-7.75, 13.25) -> (-8.75, 14.25) centre (-8.75, 13.25) ccw
  line L4 (7.75, -13.25) -> (7.75, -7.25)
  arc A11 (8.75, -6.25) -> (7.75, -7.25) centre (8.75, -7.25) ccw
  line L5 (8.75, -6.25) -> (18.75, -6.25)
  arc A12 (19.75, -7.25) -> (18.75, -6.25) centre (18.75, -7.25) ccw
  line L6 (19.75, -7.25) -> (19.75, -13.25)
  arc A13 (18.75, -14.25) -> (19.75, -13.25) centre (18.75, -13.25) ccw
  line L7 (18.75, -14.25) -> (8.75, -14.25)
  arc A14 (7.75, -13.25) -> (8.75, -14.25) centre (8.75, -13.25) ccw
  circle A15 centre (-33.8506, -28.3482) radius 1.75
  circle A16 centre (0, 0) radius 62
  line L8 (29.55, -18.55) -> (31.95, -18.55)
  line L9 (31.95, -18.55) -> (31.95, -22.95)
  line L10 (31.95, -22.95) -> (29.55, -22.95)
  line L11 (29.55, -22.95) -> (29.55, -18.55)
  circle A17 centre (31.4571, -7.9571) radius 1.5
  line L12 (-29.55, 18.55) -> (-31.95, 18.55)
  line L13 (-31.95, 18.55) -> (-31.95, 22.95)
  line L14 (-31.95, 22.95) -> (-29.55, 22.95)
  line L15 (-29.55, 22.95) -> (-29.55, 18.55)
  line L16 (6.25, 8.75) -> (6.25, 18.75)
  arc A18 (7.25, 19.75) -> (6.25, 18.75) centre (7.25, 18.75) ccw
  line L17 (7.25, 19.75) -> (13.25, 19.75)
  arc A19 (14.25, 18.75) -> (13.25, 19.75) centre (13.25, 18.75) ccw
  line L18 (14.25, 18.75) -> (14.25, 8.75)
  arc A20 (13.25, 7.75) -> (14.25, 8.75) centre (13.25, 8.75) ccw
  line L19 (13.25, 7.75) -> (7.25, 7.75)
  arc A21 (6.25, 8.75) -> (7.25, 7.75) centre (7.25, 8.75) ccw
  circle A22 centre (-28.3482, 33.8506) radius 1.75
  line L20 (-13.25, -7.75) -> (-7.25, -7.75)
  arc A23 (-6.25, -8.75) -> (-7.25, -7.75) centre (-7.25, -8.75) ccw
  line L21 (-6.25, -8.75) -> (-6.25, -18.75)
  arc A24 (-7.25, -19.75) -> (-6.25, -18.75) centre (-7.25, -18.75) ccw
  line L22 (-7.25, -19.75) -> (-13.25, -19.75)
  arc A25 (-14.25, -18.75) -> (-13.25, -19.75) centre (-13.25, -18.75) ccw
  line L23 (-14.25, -18.75) -> (-14.25, -8.75)
  arc A26 (-13.25, -7.75) -> (-14.25, -8.75) centre (-13.25, -8.75) ccw
  circle A27 centre (-31.4571, 7.9571) radius 1.5
  line L24 (22.95, 29.55) -> (18.55, 29.55)
  line L25 (18.55, 29.55) -> (18.55, 31.95)
  line L26 (18.55, 31.95) -> (22.95, 31.95)
  line L27 (22.95, 31.95) -> (22.95, 29.55)
  line L28 (-18.55, -29.55) -> (-18.55, -31.95)
  line L29 (-18.55, -31.95) -> (-22.95, -31.95)
  line L30 (-22.95, -31.95) -> (-22.95, -29.55)
  line L31 (-22.95, -29.55) -> (-18.55, -29.55)
  circle A28 centre (-7.9571, -31.4571) radius 1.5
  circle A29 centre (7.9571, 31.4571) radius 1.5
  circle A30 centre (33.8506, 28.3482) radius 1.75
  circle A31 centre (-40.8377, -37.077) radius 1.5
  circle A32 centre (-37.077, 40.8377) radius 1.5
  circle A33 centre (37.077, -40.8377) radius 1.5
  circle A34 centre (40.8377, 37.077) radius 1.5
delete_face "DeleteFace2" 1 faces at (-13.0084, -0.5308, 2)
delete_face "DeleteFace3" 1 faces at (-0.049, 12.6228, 2)
delete_face "DeleteFace4" 1 faces at (11.7995, 0.4149, 2)
delete_face "DeleteFace5" 1 faces at (-0.0967, -11.7953, 2)
delete_face "DeleteFace6" 1 faces at (1.8661, 1.4252, 2)
